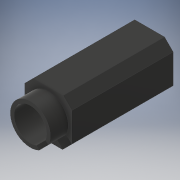
# Autodesk Inventor part: conduit_endcap
Saved by Autodesk Inventor 2017 (Build 210142000, 142)
## iProperties
Created: 2018-11-30
Part Number: conduit_endcap
Material: UHMW, Black
Document SubType Name: Modeling
Designer: ddeboer
Density: 0.94 g/cm^3
Appearance: Smooth - Black
Author: ddeboer
Autodesk Inventor part; units mm, degrees
ref_plane "YZ Plane" through (0, 0, 0) normal (1, 0, 0) x (0, 1, 0)
ref_plane "XZ Plane" through (0, 0, 0) normal (0, 1, 0) x (-1, 0, 0)
ref_plane "XY Plane" through (0, 0, 0) normal (0, 0, 1) x (1, 0, 0)
sketch "Sketch1" plane through (0, 0, 0) normal (0, 0, 1) x (1, 0, 0)
  line L0 (-12.5, -19.75) -> (12.5, -19.75)
  line L1 (19.75, -12.5) -> (19.75, 12.5)
  line L2 (12.5, 19.75) -> (-12.5, 19.75)
  line L3 (-19.75, 12.5) -> (-19.75, -12.5)
  line L4 (19.75, 19.75) -> (19.75, 19.75)
  line L5 (19.75, 19.75) -> (19.75, 19.75)
  line L6 (19.75, -12.5) -> (19.75, -12.5)
  line L7 (-12.5, -19.75) -> (-19.75, -12.5)
  line L8 (-19.75, 12.5) -> (-12.5, 19.75)
  line L9 (12.5, 19.75) -> (19.75, 12.5)
  line L10 (19.75, -12.5) -> (12.5, -19.75)
  line L11 (-19.75, 0) -> (19.75, 0) construction
  circle A0 centre (0, 0) radius 10
  point P0 (19.75, 19.75)
  point P1 (19.75, -19.75)
  point P2 (-19.75, 19.75)
  dimension "d33" = 39.5
  dimension "d34" = 39.5
  dimension "d35" = 20
  constraints: 24 end point, 10 point on line, 3 midpoint, 2 parallel, 1 centre point, 1 horizontal, 1 perpendicular
  measures "d33" distance of point (-19.75, 19.75) point (19.75, 19.75)
  measures "d34" distance of point (19.75, 19.75) point (19.75, -19.75)
  measures "d35" diameter of A0
extrude "Extrusion7" add sketch "Sketch1" along normal blind 100
sketch "Sketch8" plane through (0, 0, 100) normal (0, 0, 1) x (1, 0, 0)
  circle A0 centre (0, 0) radius 13.75
  dimension "d38" = 27.5
  constraints: 1 centre point, 1 coincident
  measures "d38" diameter of A0
extrude "Extrusion8" cut sketch "Sketch8" against normal blind 100
sketch "Sketch10" plane through (0, 0, 0) normal (0, 0, -1) x (-1, 0, 0)
  circle A0 centre (0, 0) radius 17
  dimension "d44" = 34
  constraints: 1 centre point, 1 coincident
  measures "d44" diameter of A0
extrude "Extrusion10" cut sketch "Sketch10" against normal blind 25
sketch "Sketch11" plane through (0, 0, 100) normal (0, 0, 1) x (1, 0, 0)
  circle A0 centre (0, 0) radius 16.75
  line L0 (39.1509, 23.8646) -> (-32.83, 23.8646)
  line L1 (-32.83, 23.8646) -> (-32.83, -25.2836)
  line L2 (-32.83, -25.2836) -> (39.1509, -25.2836)
  line L3 (39.1509, -25.2836) -> (39.1509, 23.8646)
  dimension "d47" = 33.5
  constraints: 8 end point, 2 parallel, 1 centre point, 1 coincident, 1 horizontal, 1 perpendicular
  measures "d47" diameter of A0
extrude "Extrusion11" cut sketch "Sketch11" against normal blind 15
sketch "Sketch12" plane through (12.5, -19.75, 85) normal (0.7071068, -0.7071068, 0) x (-0.7071068, -0.7071068, 0)
  line L0 (-10.6265, 85) -> (0.3735, 85)
  line L1 (0.3735, 85) -> (0.3735, -33.4393)
  line L2 (0.3735, -33.4393) -> (-10.6265, -33.4393)
  line L3 (-10.6265, -33.4393) -> (-10.6265, 85)
  line L4 (-5.1265, 85) -> (-5.1265, -33.4393) construction
  line L5 (0, 85) -> (-10.253, 85) projected
  point P0 (-5.1265, 85)
  dimension "d50" = 11
  constraints: 10 end point, 3 midpoint, 2 parallel, 1 horizontal, 1 perpendicular
  measures "d50" distance of L1.end L2.end
extrude "Extrusion12" cut sketch "Sketch12" against normal blind 20
body "Solid2"
